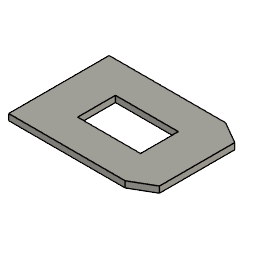
lidar_chassis (Autodesk Fusion 360 design; units mm, degrees)
part number: 2026-06-29-20-04-35-290
Autodesk Fusion 360 part; units mm, degrees
derive "DerivedContext1"
sketch "Sketch1" plane through (0, 0, 0) normal (0, 0, 1) x (1, 0, 0)
  line L0 (0, 0) -> (92.6795, 0)
  line L1 (110, 10) -> (110, 70)
  line L2 (92.6795, 80) -> (0, 80)
  line L3 (0, 80) -> (0, 0)
  line L4 (92.6795, 80) -> (110, 70)
  line L5 (92.6795, 0) -> (110, 10)
  dimension "d1" = 80
  dimension "d2" = 110
  dimension "d9" = 60
  dimension "d10" = 150
  dimension "d11" = 150
  constraint horizontal L0
  constraint vertical L1
  constraint horizontal L2
  constraint vertical L3
  constraint coincident L0.start L3.end
  measures "d1" distance of L0.start L2.end
  measures "d2" distance of L1 L3
  measures "d9" distance of L1.end L1.start
  measures "d10" angle of L2 L4
  measures "d11" angle of L0 L5
extrude "Extrude1" add sketch "Sketch1" along normal blind 5
sketch "Sketch3" plane through (0, 0, 5) normal (0, 0, 1) x (-1, 0, 0)
  line L0 (-92.6795, -80) -> (0, -80)
  line L1 (0, -80) -> (0, 0)
  line L2 (0, 0) -> (-92.6795, 0)
  line L3 (-92.6795, 0) -> (-110, -10)
  line L4 (-110, -10) -> (-110, -70)
  line L5 (-110, -70) -> (-92.6795, -80)
  line L6 (-80, -25) -> (-30, -25)
  line L7 (-30, -25) -> (-30, -55)
  line L8 (-30, -55) -> (-80, -55)
  line L9 (-80, -55) -> (-80, -25)
  dimension "d23" = 30
  dimension "d24" = 50
  dimension "d25" = 25
  dimension "d26" = 30
  constraint horizontal L6
  constraint vertical L7
  constraint horizontal L8
  constraint vertical L9
  measures "d23" distance of L6.end L7.end
  measures "d24" distance of L6.start L6.end
  measures "d25" distance of L2 L6
  measures "d26" distance of L1 L7
extrude "Extrude2" cut sketch "Sketch3" against normal through all contours L6 L7 L8 L9
